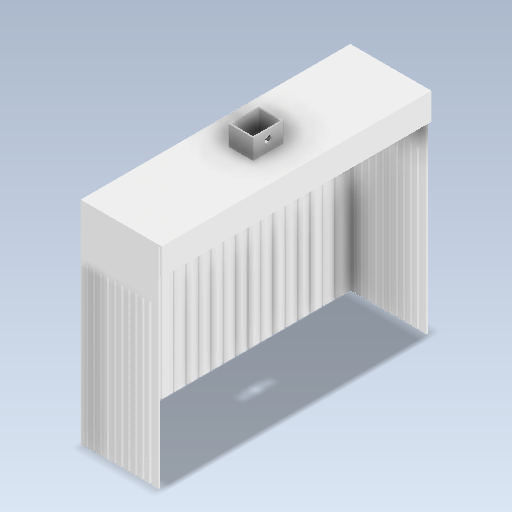
# Autodesk Inventor part: Sensors Holder V3
Saved by Autodesk Inventor 2020 (Build 240168000, 168)
## iProperties
Created: 2020-08-10
Part Number: Sensors Holder V3
Material: Generic
Document SubType Name: Modeling
Designer: Abbas
Density: 1 g/cm^3
Appearance: Default
Author: Abbas
Autodesk Inventor part; units mm, degrees
ref_plane "YZ Plane" through (0, 0, 0) normal (1, 0, 0) x (0, 1, 0)
ref_plane "XZ Plane" through (0, 0, 0) normal (0, 1, 0) x (-1, 0, 0)
sketch "Sketch1" plane through (0, 0, 0) normal (0, 1, 0) x (-1, 0, 0)
  line L0 (75, 250) -> (-75, 250)
  line L1 (-75, 250) -> (-75, -250)
  line L2 (-75, -250) -> (75, -250)
  line L3 (75, -250) -> (75, 250)
  line L4 (75, 250) -> (-75, -250) construction
  line L5 (-75, 250) -> (75, -250) construction
  line L6 (-72, 250) -> (-75, 250)
  line L7 (-75, 250) -> (-75, -250)
  line L8 (-75, -250) -> (-72, -250)
  line L9 (-72, -250) -> (-72, 250)
  line L10 (-72, 250) -> (-75, -250) construction
  line L11 (-75, 250) -> (-72, -250) construction
  line L12 (75, 250) -> (-69, 250)
  line L13 (-69, 250) -> (-69, 247)
  line L14 (-69, 247) -> (75, 247)
  line L15 (75, 247) -> (75, 250)
  line L16 (75, 250) -> (-69, 247) construction
  line L17 (-69, 250) -> (75, 247) construction
  line L18 (75, -247) -> (-69, -247)
  line L19 (-69, -247) -> (-69, -250)
  line L20 (-69, -250) -> (75, -250)
  line L21 (75, -250) -> (75, -247)
  line L22 (75, -247) -> (-69, -250) construction
  line L23 (-69, -247) -> (75, -250) construction
  line L24 (75, 247) -> (72, 247)
  line L25 (72, 247) -> (72, -247)
  line L26 (72, -247) -> (75, -247)
  line L27 (75, -247) -> (75, 247)
  line L28 (75, 247) -> (72, -247) construction
  line L29 (72, 247) -> (75, -247) construction
  point P0 (0, 0)
  point P1 (-73.5, 0)
  point P2 (-75, 0)
  point P3 (3, 248.5)
  point P4 (3, -248.5)
  point P5 (73.5, 0)
  point P6 (75, 0)
  point P7 (72, -247)
  point P8 (72, 247)
  point P9 (-69, 250)
  point P10 (-69, -250)
  point P11 (75, -247)
  point P12 (75, -247)
  point P13 (75, 247)
  point P14 (75, 247)
  point P15 (75, -247)
  point P16 (75, 247)
  dimension "d0" = 150
  dimension "d1" = 500
  dimension "d2" = 3
  dimension "d3" = 500
  dimension "d4" = 144
  dimension "d5" = 3
  dimension "d6" = 144
  dimension "d7" = 3
  dimension "d8" = 3
  dimension "d9" = 494
  constraints: 60 end point, 14 midpoint, 10 parallel, 5 horizontal, 5 perpendicular
  measures "d0" distance of L2.end L1.end
  measures "d1" distance of L1.end L0.end
  measures "d2" distance of L8.end L7.end
  measures "d3" distance of L7.end L6.end
  measures "d4" distance of L14.end L13.end
  measures "d5" distance of L13.end L12.end
  measures "d6" distance of L2.end L19.end
  measures "d7" distance of L19.end L18.end
  measures "d8" distance of L26.end L25.end
  measures "d9" distance of L25.end L24.end
extrude "Extrusion1" add sketch "Sketch1" against normal blind 3 contours L3 L14 L13 L0 | L13 L14 L25 L18 L19 L2 L9 L0 | L9 L2 L1 L0 | L3 L2 L19 L18
extrude "Extrusion2" add sketch "Sketch1" against normal blind 50 contours L9 L2 L1 L0
extrude "Extrusion3" add sketch "Sketch1" against normal blind 393 contours L3 L14 L13 L0 | L3 L18 L25 L14 | L3 L2 L19 L18
sketch "Sketch2" plane through (0, 0, 0) normal (0, 1, 0) x (1, 0, 0)
  circle A0 centre (0, -12.655) radius 8.2
  circle A1 centre (0, 12.655) radius 8.2
  line L0 (-6.0435, -5.9922) -> (-10.65, -5.9922)
  line L1 (-10.65, -5.9922) -> (-10.65, 6.0078)
  line L2 (-10.65, 6.0078) -> (-6.0435, 6.0078)
  line L3 (-6.0435, 6.0078) -> (-6.0435, -5.9922)
  line L4 (-6.0435, -5.9922) -> (-10.65, 6.0078) construction
  line L5 (-10.65, -5.9922) -> (-6.0435, 6.0078) construction
  line L6 (0, 12.655) -> (0, -12.655)
  point P0 (0, 0)
  point P1 (0, 0)
  point P2 (-8.3467, 0.0078)
  point P3 (0, 0)
  dimension "d16" = 16.4
  dimension "d17" = 16.4
  dimension "d18" = 25.31
  dimension "d19" = 4.6065
  dimension "d20" = 12
  dimension "d21" = 12.6628
  dimension "d22" = 8.3467
  constraints: 14 end point, 3 midpoint, 2 centre point, 2 parallel, 1 coincident, 1 horizontal, 1 perpendicular, 1 vertical
  measures "d16" diameter of A0
  measures "d17" diameter of A1
  measures "d18" distance of L6.start L6.end
  measures "d19" distance of L1.end L2.end
  measures "d20" distance of L0.end L1.end
  measures "d21" vertical distance of point (-8.347, 0.008) L6.end
  measures "d22" horizontal distance of L6.end point (-8.347, 0.008)
extrude "Extrusion4" cut sketch "Sketch2" along normal mid plane 10
ref_plane "Work Plane2" through (-1.5, -393, 247) normal (1, 0, 0) x (0, 0, -1)
sketch "Sketch4" plane through (-1.5, -393, 247) normal (1, 0, 0) x (0, 0, -1)
  line L0 (247, 390) -> (50.5, 49.652)
  line L1 (247, 390) -> (640, 390) construction
  line L2 (247, 390) -> (443.5, 49.652)
  line L3 (247, 390) -> (640, 390) construction
  line L4 (247, 390) -> (247, -3)
  line L5 (247, 390) -> (640, 390) construction
  line L6 (0, 390) -> (0, 0) projected
  line L7 (0, -37.8165) -> (497, -43.0127)
  line L8 (497, 393) -> (497, 0) projected
  line L9 (242.545, 390) -> (226.145, 390) projected
  line L10 (267.855, 390) -> (251.455, 390) projected
  line L11 (242.545, 390) -> (251.455, 390)
  point P0 (247, 393)
  dimension "d35" = 393
  dimension "d36" = 120
  dimension "d37" = 393
  dimension "d38" = 60
  dimension "d39" = 393
  dimension "d40" = 90
  constraints: 16 end point, 4 point on line, 3 equal length, 3 horizontal, 1 collinear, 1 midpoint, 1 vertical
  measures "d35" distance of L0.start L0.end
  measures "d36" angle of L0 L1
  measures "d37" distance of L0.start L2.end
  measures "d38" angle of L2 L3
  measures "d39" distance of L0.start L4.end
  measures "d40" angle of L4 L5
sketch "Sketch5" plane through (-75, 0, 250) normal (0, 0, 1) x (1, 0, 0)
  line L0 (10.5, -100) -> (13.5, -100)
  line L1 (13.5, -100) -> (13.5, -393)
  line L2 (13.5, -393) -> (10.5, -393)
  line L3 (10.5, -393) -> (10.5, -100)
  line L4 (144, -393) -> (0, -393) projected
  line L5 (0, 0) -> (0, -393) projected
  line L6 (26.5, -100) -> (26.5, -393)
  line L7 (23.5, -393) -> (23.5, -100)
  line L8 (23.5, -100) -> (26.5, -100)
  line L9 (26.5, -393) -> (23.5, -393)
  line L10 (39.5, -100) -> (39.5, -393)
  line L11 (36.5, -393) -> (36.5, -100)
  line L12 (36.5, -100) -> (39.5, -100)
  line L13 (39.5, -393) -> (36.5, -393)
  line L14 (52.5, -100) -> (52.5, -393)
  line L15 (49.5, -393) -> (49.5, -100)
  line L16 (49.5, -100) -> (52.5, -100)
  line L17 (52.5, -393) -> (49.5, -393)
  line L18 (65.5, -100) -> (65.5, -393)
  line L19 (62.5, -393) -> (62.5, -100)
  line L20 (62.5, -100) -> (65.5, -100)
  line L21 (65.5, -393) -> (62.5, -393)
  line L22 (78.5, -100) -> (78.5, -393)
  line L23 (75.5, -393) -> (75.5, -100)
  line L24 (75.5, -100) -> (78.5, -100)
  line L25 (78.5, -393) -> (75.5, -393)
  line L26 (91.5, -100) -> (91.5, -393)
  line L27 (88.5, -393) -> (88.5, -100)
  line L28 (88.5, -100) -> (91.5, -100)
  line L29 (91.5, -393) -> (88.5, -393)
  line L30 (104.5, -100) -> (104.5, -393)
  line L31 (101.5, -393) -> (101.5, -100)
  line L32 (101.5, -100) -> (104.5, -100)
  line L33 (104.5, -393) -> (101.5, -393)
  line L34 (117.5, -100) -> (117.5, -393)
  line L35 (114.5, -393) -> (114.5, -100)
  line L36 (114.5, -100) -> (117.5, -100)
  line L37 (117.5, -393) -> (114.5, -393)
  line L38 (130.5, -100) -> (130.5, -393)
  line L39 (127.5, -393) -> (127.5, -100)
  line L40 (127.5, -100) -> (130.5, -100)
  line L41 (130.5, -393) -> (127.5, -393)
  point P0 (75, 0)
  point P1 (12, -393)
  point P2 (25, -393)
  point P3 (38, -393)
  point P4 (51, -393)
  point P5 (64, -393)
  point P6 (77, -393)
  point P7 (90, -393)
  point P8 (103, -393)
  point P9 (116, -393)
  point P10 (129, -393)
  dimension "d41" = 3
  dimension "d42" = 293
  dimension "d43" = 10.5
  dimension "d46" = 13
  constraints: 80 end point, 2 horizontal, 2 parallel, 1 midpoint, 1 perpendicular, 1 point on line, 81 other
  measures "d41" distance of L1.end L2.end
  measures "d42" distance of L0.end L1.end
  measures "d43" distance between parallel lines of L5 L3
  measures "d46" distance of L0.end L6.start
extrude "Extrusion5" cut sketch "Sketch5" against normal blind 600
sketch "Sketch6" plane through (-75, 0, -250) normal (-1, 0, 0) x (0, 0, 1)
  line L0 (30, -100) -> (33, -100)
  line L1 (33, -100) -> (33, -393)
  line L2 (33, -393) -> (30, -393)
  line L3 (30, -393) -> (30, -100)
  line L4 (500, -393) -> (0, -393) projected
  line L5 (0, 0) -> (0, -393) projected
  line L6 (53, -100) -> (56, -100)
  line L7 (56, -100) -> (56, -393)
  line L8 (53, -393) -> (53, -100)
  line L9 (76, -100) -> (79, -100)
  line L10 (79, -100) -> (79, -393)
  line L11 (76, -393) -> (76, -100)
  line L12 (99, -100) -> (102, -100)
  line L13 (102, -100) -> (102, -393)
  line L14 (99, -393) -> (99, -100)
  line L15 (122, -100) -> (125, -100)
  line L16 (125, -100) -> (125, -393)
  line L17 (122, -393) -> (122, -100)
  line L18 (145, -100) -> (148, -100)
  line L19 (148, -100) -> (148, -393)
  line L20 (145, -393) -> (145, -100)
  line L21 (168, -100) -> (171, -100)
  line L22 (171, -100) -> (171, -393)
  line L23 (168, -393) -> (168, -100)
  line L24 (191, -100) -> (194, -100)
  line L25 (194, -100) -> (194, -393)
  line L26 (191, -393) -> (191, -100)
  line L27 (214, -100) -> (217, -100)
  line L28 (217, -100) -> (217, -393)
  line L29 (214, -393) -> (214, -100)
  line L30 (237, -100) -> (240, -100)
  line L31 (240, -100) -> (240, -393)
  line L32 (237, -393) -> (237, -100)
  line L33 (260, -100) -> (263, -100)
  line L34 (263, -100) -> (263, -393)
  line L35 (260, -393) -> (260, -100)
  line L36 (283, -100) -> (286, -100)
  line L37 (286, -100) -> (286, -393)
  line L38 (283, -393) -> (283, -100)
  line L39 (306, -100) -> (309, -100)
  line L40 (309, -100) -> (309, -393)
  line L41 (306, -393) -> (306, -100)
  line L42 (329, -100) -> (332, -100)
  line L43 (332, -100) -> (332, -393)
  line L44 (329, -393) -> (329, -100)
  line L45 (352, -100) -> (355, -100)
  line L46 (355, -100) -> (355, -393)
  line L47 (352, -393) -> (352, -100)
  line L48 (375, -100) -> (378, -100)
  line L49 (378, -100) -> (378, -393)
  line L50 (375, -393) -> (375, -100)
  line L51 (398, -100) -> (401, -100)
  line L52 (401, -100) -> (401, -393)
  line L53 (398, -393) -> (398, -100)
  line L54 (421, -100) -> (424, -100)
  line L55 (424, -100) -> (424, -393)
  line L56 (421, -393) -> (421, -100)
  line L57 (444, -100) -> (447, -100)
  line L58 (447, -100) -> (447, -393)
  line L59 (444, -393) -> (444, -100)
  line L60 (467, -100) -> (470, -100)
  line L61 (470, -100) -> (470, -393)
  line L62 (467, -393) -> (467, -100)
  point P0 (250, 0)
  point P1 (31.5, -393)
  point P2 (56, -393)
  dimension "d53" = 3
  dimension "d54" = 293
  dimension "d55" = 30
  dimension "d58" = 23
  constraints: 122 end point, 76 horizontal alignment, 40 parallel, 19 collinear, 1 horizontal, 1 midpoint, 1 perpendicular, 2 other
  measures "d53" distance of L1.end L2.end
  measures "d54" distance of L0.end L1.end
  measures "d55" distance between parallel lines of L5 L3
  measures "d58" distance of L0.start L6.start
extrude "Extrusion6" cut sketch "Sketch6" against normal blind 20
sketch "Sketch7" plane through (0, 0, 0) normal (0, 1, 0) x (1, 0, 0)
  line L0 (-20, -25) -> (20, -25)
  line L1 (20, -25) -> (20, 25)
  line L2 (20, 25) -> (-20, 25)
  line L3 (-20, 25) -> (-20, -25)
  line L4 (-20, -25) -> (20, 25) construction
  line L5 (20, -25) -> (-20, 25) construction
  line L6 (-23, -28) -> (23, -28)
  line L7 (23, -28) -> (23, 28)
  line L8 (23, 28) -> (-23, 28)
  line L9 (-23, 28) -> (-23, -28)
  line L10 (-23, -28) -> (23, 28) construction
  line L11 (23, -28) -> (-23, 28) construction
  point P0 (0, 0)
  dimension "d65" = 40
  dimension "d66" = 50
  dimension "d67" = 46
  dimension "d68" = 56
  constraints: 24 end point, 4 midpoint, 4 parallel, 2 horizontal, 2 perpendicular
  measures "d65" distance of L2.end L1.end
  measures "d66" distance of L1.end L0.end
  measures "d67" distance of L8.end L7.end
  measures "d68" distance of L7.end L6.end
extrude "Extrusion7" add sketch "Sketch7" along normal blind 37
sketch "Sketch9" plane through (23, 0, 28) normal (1, 0, 0) x (0, 0, -1)
  circle A0 centre (28, 20) radius 6.5
  point P0 (28, 0)
  dimension "d75" = 13
  constraints: 1 centre point
  measures "d75" diameter of A0
extrude "Extrusion9" cut sketch "Sketch9" against normal blind 10
body "Solid1"
